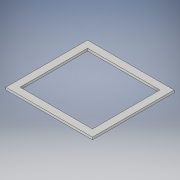
# Autodesk Inventor part: Scannerframetop
Saved by Autodesk Inventor 2019 (Build 230136000, 136)
## iProperties
Created: 2018-10-07
Part Number: Scannerframetop
Material: Generic
Document SubType Name: Modeling
Designer: paperspace
Density: 1 g/cm^3
Appearance: Default
Author: paperspace
Autodesk Inventor part; units mm, degrees
ref_plane "YZ Plane" through (0, 0, 0) normal (1, 0, 0) x (0, 1, 0)
ref_plane "XZ Plane" through (0, 0, 0) normal (0, 1, 0) x (-1, 0, 0)
ref_plane "XY Plane" through (0, 0, 0) normal (0, 0, 1) x (1, 0, 0)
sketch "Sketch1" plane through (0, 0, 0) normal (0, 1, 0) x (-1, 0, 0)
  line L0 (0, 0) -> (71, 0)
  line L1 (71, 0) -> (71, -67)
  line L2 (71, -67) -> (0, -67)
  line L3 (0, -67) -> (0, 0)
  line L4 (65.2, -61.2) -> (65.2, -5.8)
  line L5 (65.2, -5.8) -> (5.8, -5.8)
  line L6 (5.8, -5.8) -> (5.8, -61.2)
  line L7 (5.8, -61.2) -> (65.2, -61.2)
  dimension "d0" = 71
  dimension "d1" = 67
  dimension "d2" = 5.8
  constraints: 16 end point, 4 parallel, 2 perpendicular, 1 horizontal, 3 other
  measures "d0" distance of L1.end L2.end
  measures "d1" distance of L0.end L1.end
  measures "d2" distance between parallel lines of L1 L4
extrude "Extrusion1" add sketch "Sketch1" along normal blind 2
body "Solid1"
